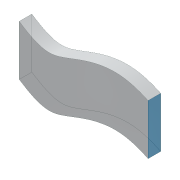
# Autodesk Inventor part: ThickThinProfile
Saved by Autodesk Inventor 2014 (Build 180170000, 170)
## iProperties
Created: 2014-12-16
Part Number: ThickThinProfile
Material: Glass
Document SubType Name: Modeling
Designer: Yogesh
Density: 2.18 g/cm^3
Appearance: Clear
Author: Yogesh
Autodesk Inventor part; units mm, degrees
ref_plane "YZ Plane" through (0, 0, 0) normal (1, 0, 0) x (0, 1, 0)
ref_plane "XZ Plane" through (0, 0, 0) normal (0, 1, 0) x (-1, 0, 0)
ref_plane "XY Plane" through (0, 0, 0) normal (0, 0, 1) x (1, 0, 0)
sketch "Sketch1" plane through (0, 0, 0) normal (0, 1, 0) x (-1, 0, 0)
  line L0 (0, 10) -> (0, -10)
  line L1 (51.1673, 11.668) -> (51.1673, -8.3082)
  line L2 (0, 10) -> (7.8343, 13.5739) construction
  line L3 (7.8343, 13.5739) -> (16.9195, 13.5739) construction
  line L4 (16.9195, 13.5739) -> (25.4703, 11.668) construction
  line L5 (25.4703, 11.668) -> (35.09, 7.0272) construction
  line L6 (35.09, 7.0272) -> (42.1712, 5.5575) construction
  line L7 (42.1712, 5.5575) -> (51.1673, 11.668) construction
  spline S0 degree 4 poles (0, 10) (7.8343, 13.5739) (16.9195, 13.5739) (25.4703, 11.668) (35.09, 7.0272) (42.1712, 5.5575) (51.1673, 11.668) knots 1 1 1 1 1 2 3 4 4 4 4 4
  line L8 (0, -10) -> (7.7654, -6.2687) construction
  line L9 (7.7654, -6.2687) -> (16.8507, -6.2687) construction
  line L10 (16.8507, -6.2687) -> (25.4015, -8.3082) construction
  line L11 (25.4015, -8.3082) -> (35.0212, -12.949) construction
  line L12 (35.0212, -12.949) -> (42.1023, -14.4187) construction
  line L13 (42.1023, -14.4187) -> (51.1673, -8.3082) construction
  spline S1 degree 4 poles (0, -10) (7.7654, -6.2687) (16.8507, -6.2687) (25.4015, -8.3082) (35.0212, -12.949) (42.1023, -14.4187) (51.1673, -8.3082) knots 1 1 1 1 1 2 3 4 4 4 4 4
  point P0 (0, 0)
  constraints: 4 end point, 2 vertical, 1 midpoint, 1 perpendicular, 6 other
extrude "Extrusion1" add sketch "Sketch1" along normal mid plane 5
body "Solid1"
